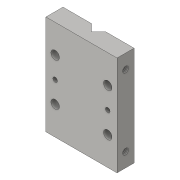
# Autodesk Inventor part: Unterstempel_2016_iLogic
Saved by Autodesk Inventor 2016 (Build 200138000, 138)
## iProperties
Created: 2015-09-08
Part Number: Unterstempel_2016_iLogic
Material: Generisch
Document SubType Name: Modeling
Designer: bauermeisterdi
Density: 1 g/cm^3
Appearance: Vorgabe
Author: bauermeisterdi
Autodesk Inventor part; units mm, degrees
ref_plane "YZ Plane" through (0, 0, 0) normal (1, 0, 0) x (0, 1, 0)
ref_plane "XZ Plane" through (0, 0, 0) normal (0, 1, 0) x (-1, 0, 0)
ref_plane "XY Plane" through (0, 0, 0) normal (0, 0, 1) x (1, 0, 0)
sketch "Skizze_Grundkörper" plane through (0, 0, 0) normal (0, 0, 1) x (1, 0, 0)
  line L0 (-25, 0) -> (25, 0)
  line L1 (25, 0) -> (25, 12)
  line L2 (25, 12) -> (5, 12)
  line L3 (-35, 0) -> (35, 0) projected
  line L4 (0, -2.4) -> (0, 14.4) projected
  line L5 (5, 12) -> (0, 7)
  line L6 (0, 7) -> (-5, 12)
  line L7 (-5, 12) -> (-25, 12)
  line L8 (-25, 12) -> (-25, 0)
  point P0 (0, 0)
  dimension "Breite" = 50
  dimension "Höhe" = 12
  dimension "Nuttiefe" = 5
  dimension "Nutwinkel" = 90
  constraints: 14 end point, 2 collinear, 2 horizontal, 2 perpendicular, 1 point on line, 2 other
  measures "Breite" distance of L0.start L0.end
  measures "Höhe" distance of L0.end L1.end
  measures "Nuttiefe" distance from line of L5.end L7
  measures "Nutwinkel" angle of L5 L6
extrude "Grundkörper" add sketch "Skizze_Grundkörper" along normal mid plane 70
sketch "Skizze_Bohrung_6H7" plane through (-25, 12, 35) normal (0, 1, 0) x (1, 0, 0)
  line L0 (-10, 35) -> (60, 35) projected
  line L1 (25, 84) -> (25, -14) projected
  point P0 (25, 35)
  point P1 (6.5, 50)
  point P2 (43.5, 50)
  point P3 (43.5, 20)
  point P4 (6.5, 20)
  dimension "Abstand_Breite_Bohrung_6H7" = 37
  dimension "Abstand_Länge_Bohrung_6H7" = 30
  constraints: 3 symmetric about line
  measures "Abstand_Breite_Bohrung_6H7" distance of point (43.5, 50) point (6.5, 50)
  measures "Abstand_Länge_Bohrung_6H7" distance of point (43.5, 50) point (43.5, 20)
hole "Bohrung_6H7" at (-18.5, 12, -15) at (18.5, 12, -15) at (18.5, 12, 15) at (-18.5, 12, 15) direction (0, -1, 0) diameter 6 end through all
sketch "Skizze_Gewinde_M4" plane through (-25, 0, 35) normal (0, -1, 0) x (1, 0, 0)
  line L0 (-10, -35) -> (60, -35) projected
  line L1 (25, -84) -> (25, 14) projected
  point P0 (25, -35)
  point P1 (6.5, -35)
  point P2 (43.5, -35)
  dimension "Abstand_Breite_Gewinde_M4" = 37
  constraints: 2 point on line, 1 symmetric about line
  measures "Abstand_Breite_Gewinde_M4" distance of point (43.5, -35) point (6.5, -35)
hole "Gewinde_M4" at (-18.5, 0, 0) at (18.5, 0, 0) direction (0, 1, 0) diameter 3.242 depth 9 tip angle 118 thread size "M4x0.7" class "6H" standard "ISO Metric profile"
sketch "Skizze_Gewinde_M5" plane through (25, 0, 35) normal (1, 0, 0) x (0, 0, -1)
  line L0 (35, -2.4) -> (35, 14.4) projected
  line L1 (84, 0) -> (-14, 0) projected
  point P0 (35, 0)
  point P1 (10, 6)
  point P2 (60, 6)
  dimension "Abstand_Länge_Gewinde_M5" = 50
  dimension "Abstand_Höhe_Gewinde_M5" = 6
  constraints: 1 symmetric about line
  measures "Abstand_Länge_Gewinde_M5" distance of point (60, 6) point (10, 6)
  measures "Abstand_Höhe_Gewinde_M5" distance from line of point (10, 6) L1
hole "Gewinde_M5" at (25, 6, 25) at (25, 6, -25) direction (-1, 0, 0) diameter 4.134 depth 16 tip angle 118 thread size "M5x0.8" class "6H" standard "ISO Metric profile"
pattern_circular "Anordnung_Gewinde_M5" count 2 over 360 about axis through (0, -10, 0) along (0, 1, 0) of "Gewinde_M5"
equation "\"Abstand_Höhe_Gewinde_M5\" = 0.5 * Höhe"
